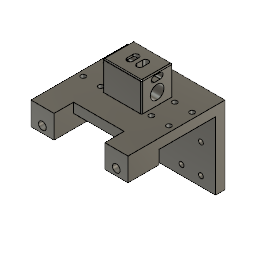
axis_connector (Autodesk Fusion 360 design; units mm, degrees)
Autodesk Fusion 360 part; units mm, degrees
note: some values were not read from the file. Chosen so that the rebuilt part matches the saved one: which bodies a step acts on.
sketch "Sketch1" plane through (0, 0, 0) normal (0, 0, 1) x (1, 0, 0)
  line L0 (0, 0) -> (100, 0)
  line L1 (100, 0) -> (100, 80)
  line L2 (100, 80) -> (0, 80)
  line L3 (0, 80) -> (0, 0)
  dimension "d1" = 80
  dimension "d2" = 100
  constraint horizontal L0
  constraint vertical L1
  constraint horizontal L2
  constraint vertical L3
  constraint coincident L0.start L3.end
  measures "d1" distance of L0.start L2.end
  measures "d2" distance of L0.start L0.end
extrude "Extrude1" add sketch "Sketch1" along normal blind 10 makes body 1
sketch "Sketch2" plane through (0, 0, 10) normal (0, 0, 1) x (-1, 0, 0)
  line L0 (0, -80) -> (0, 0)
  line L1 (0, 0) -> (-100, 0)
  line L2 (-100, 0) -> (-100, -80)
  line L3 (-100, -80) -> (0, -80)
  line L4 (-30, -40) -> (-30, -55.875)
  line L5 (-30, -55.875) -> (0, -55.875)
  line L6 (0, -55.875) -> (0, -40)
  line L7 (-30.0062, -40) -> (-30.0062, -24.125)
  line L8 (-30.0062, -24.125) -> (0, -24.125)
  line L9 (0, -24.125) -> (0, -40)
  line L10 (-70, -40) -> (-70, -55.875)
  line L11 (-70, -55.875) -> (-100, -55.875)
  line L12 (-100, -55.875) -> (-100, -40)
  line L13 (-70, -40) -> (-70, -24.125)
  line L14 (-70, -24.125) -> (-100, -24.125)
  line L15 (-100, -24.125) -> (-100, -40)
  line L16 (0, -40) -> (-30, -40)
  line L17 (-30, -40) -> (-30, -28)
  line L18 (0, -28) -> (0, -40)
  line L19 (0, -40) -> (-30, -40)
  line L20 (-30, -40) -> (-30, -52)
  line L21 (0, -52) -> (0, -40)
  line L22 (-6, -54.5) -> (-6, -55.875)
  line L23 (-24, -54.5) -> (-24, -55.875)
  circle A0 centre (-6, -52) radius 2.5
  circle A1 centre (-24, -52) radius 2.5
  line L24 (-6, -25.5) -> (-6, -24.125)
  line L25 (-24.0062, -25.5) -> (-24.0062, -24.125)
  circle A2 centre (-6, -28) radius 2.5
  circle A3 centre (-24.0062, -28) radius 2.5
  line L26 (-30, -28) -> (-26.5062, -28)
  line L27 (-21.5062, -28) -> (-8.5, -28)
  line L28 (-3.5, -28) -> (0, -28)
  line L29 (-3.5, -52) -> (0, -52)
  line L30 (-30, -52) -> (-26.5, -52)
  line L31 (-21.5, -52) -> (-8.5, -52)
  line L32 (-100, -40) -> (-70, -40)
  line L33 (-70, -40) -> (-70, -52)
  line L34 (-100, -52) -> (-100, -40)
  line L35 (-100, -40) -> (-70, -40)
  line L36 (-70, -40) -> (-70, -28)
  line L37 (-100, -28) -> (-100, -40)
  line L38 (-76, -25.5079) -> (-76, -24.125)
  line L39 (-94, -25.5) -> (-94, -24.125)
  line L40 (-76, -54.5) -> (-76, -55.875)
  line L41 (-94, -54.5) -> (-94, -55.875)
  circle A4 centre (-94, -28) radius 2.5
  circle A5 centre (-76, -52) radius 2.5
  circle A6 centre (-94, -52) radius 2.5
  line L42 (-70, -28) -> (-73.6983, -28)
  line L43 (-78.6983, -28) -> (-91.5, -28)
  line L44 (-96.5, -28) -> (-100, -28)
  line L45 (-70, -52) -> (-73.5, -52)
  line L46 (-78.5, -52) -> (-91.5, -52)
  line L47 (-96.5, -52) -> (-100, -52)
  line L48 (-30, -40) -> (-70, -40)
  line L49 (-78.5, -28) -> (-78.6983, -28)
  circle A7 centre (-76, -28) radius 2.5
  line L50 (-30, -24) -> (-70, -24)
  line L51 (-70, -24) -> (-70, -56)
  line L52 (-70, -56) -> (-30, -56)
  line L53 (-30, -56) -> (-30, -24)
  line L54 (-30, -24) -> (-70, -56) construction
  line L55 (-70, -24) -> (-30, -56) construction
  point P0 (0, -40)
  point P1 (-100, -40)
  point P2 (-50, -40)
  point P3 (-50, -40)
  dimension "d5" = 15.875
  dimension "d6" = 30
  dimension "d7" = 15.875
  dimension "d8" = 30
  dimension "d9" = 15.875
  dimension "d10" = 15.875
  dimension "d11" = 30
  dimension "d12" = 12
  dimension "d13" = 12
  dimension "d15" = 6
  dimension "d16" = 6
  dimension "d17" = 5
  dimension "d18" = 5
  dimension "d19" = 6
  dimension "d20" = 6
  dimension "d21" = 5
  dimension "d22" = 5
  dimension "d24" = 12
  dimension "d25" = 30
  dimension "d26" = 12
  dimension "d27" = 6
  dimension "d28" = 6
  dimension "d29" = 6
  dimension "d30" = 6
  dimension "d32" = 5
  dimension "d33" = 5
  dimension "d34" = 5
  dimension "d35" = 30
  dimension "d36" = 5
  dimension "d37" = 32
  dimension "d38" = 40
  constraint midpoint L0 P0
  constraint midpoint L2 P1
  constraint vertical L4
  constraint horizontal L5
  constraint vertical L6
  constraint coincident P0 L6.end
  constraint vertical L7
  constraint horizontal L8
  constraint vertical L9
  constraint vertical L10
  constraint horizontal L11
  constraint vertical L12
  constraint coincident P1 L12.end
  constraint vertical L13
  constraint horizontal L14
  constraint vertical L15
  constraint horizontal L16
  constraint vertical L17
  constraint horizontal L26
  constraint vertical L18
  constraint horizontal L19
  constraint vertical L20
  constraint horizontal L30
  constraint vertical L21
  constraint coincident L5 L22.end
  constraint perpendicular L5 L22
  constraint coincident L5 L23.end
  constraint perpendicular L5 L23
  constraint coincident L8 L24.end
  constraint perpendicular L8 L24
  constraint coincident L8 L25.end
  constraint perpendicular L8 L25
  constraint coincident A2 L24.start
  constraint coincident A3 L25.start
  constraint coincident A3 L26.end
  constraint coincident A3 L27.start
  constraint collinear L26 L27
  constraint coincident A2 L27.end
  constraint coincident A2 L28.start
  constraint collinear L27 L28
  constraint coincident A0 L29.start
  constraint collinear L29 L30
  constraint coincident A0 L31.end
  constraint coincident A0 L22.start
  constraint coincident A1 L31.start
  constraint collinear L30 L31
  constraint coincident A1 L30.end
  constraint coincident A1 L23.start
  constraint horizontal L32
  constraint vertical L33
  constraint horizontal L45
  constraint vertical L34
  constraint horizontal L35
  constraint vertical L36
  constraint horizontal L42
  constraint vertical L37
  constraint coincident L14 L38.end
  constraint perpendicular L14 L38
  constraint coincident L14 L39.end
  constraint perpendicular L14 L39
  constraint coincident L11 L40.end
  constraint perpendicular L11 L40
  constraint coincident L11 L41.end
  constraint perpendicular L11 L41
  constraint collinear L42 L43
  constraint coincident A4 L43.end
  constraint collinear L43 L44
  constraint coincident A4 L39.start
  constraint coincident A4 L44.start
  constraint coincident A5 L45.end
  constraint collinear L45 L46
  constraint coincident A5 L40.start
  constraint coincident A5 L46.start
  constraint coincident A6 L46.end
  constraint collinear L46 L47
  constraint coincident A6 L41.start
  constraint coincident A6 L47.start
  constraint perpendicular L36 L48
  constraint parallel L43 L49
  constraint coincident A7 L49.start
  constraint midpoint L48 P3
  constraint perpendicular L50 L51
  constraint parallel L50 L52
  constraint parallel L51 L53
  constraint horizontal L50
  constraint coincident L54 P3
  constraint coincident L55 P3
  constraint coincident P3 P2
  measures "d5" distance of P0 L5.end
  measures "d6" distance of P0 L4.start
  measures "d7" distance of P0 L8.end
  measures "d8" distance of P1 L10.start
  measures "d9" distance of P1 L11.end
  measures "d10" distance of P1 L14.end
  measures "d11" distance of P0 L4.start
  measures "d12" distance of P0 L18.start
  measures "d13" distance of P0 L21.start
  measures "d15" distance of L6 L22
  measures "d16" distance of L4 L23
  measures "d17" diameter of A0
  measures "d18" diameter of A1
  measures "d19" distance of L9 L24
  measures "d20" distance of L7 L25
  measures "d21" diameter of A2
  measures "d22" diameter of A3
  measures "d24" distance of P1 L34.start
  measures "d25" distance of P1 L10.start
  measures "d26" distance of P1 L37.start
  measures "d27" distance of L10 L40
  measures "d28" distance of L12 L41
  measures "d29" distance of L13 L38
  measures "d30" distance of L15 L39
  measures "d32" diameter of A4
  measures "d33" diameter of A5
  measures "d34" diameter of A6
  measures "d35" distance of L13 L37
  measures "d36" diameter of A7
  measures "d37" distance of L50.end L51.end
  measures "d38" distance of L51.end L52.end
extrude "Extrude2" cut sketch "Sketch2" against normal blind 10 contours A0 | A1 | A6 | A2 | A5 | A3 | A4 | A7 bodies 1
sketch "Sketch3" plane through (0, 0, 10) normal (0, 0, 1) x (-1, 0, 0)
  circle A0 centre (-94, -52) radius 2.5
  circle A1 centre (-24.0062, -28) radius 2.5
  circle A2 centre (-6, -28) radius 2.5
  circle A3 centre (-76, -28) radius 2.5
  circle A4 centre (-76, -52) radius 2.5
  circle A5 centre (-24, -52) radius 2.5
  circle A6 centre (-6, -52) radius 2.5
  circle A7 centre (-94, -28) radius 2.5
  line L0 (0, -80) -> (0, 0)
  line L1 (0, 0) -> (-100, 0)
  line L2 (-100, 0) -> (-100, -80)
  line L3 (-100, -80) -> (0, -80)
  line L4 (-70, -56) -> (-30, -56)
  line L5 (-30, -56) -> (-30, -24)
  line L6 (-30, -24) -> (-70, -24)
  line L7 (-70, -24) -> (-70, -56)
  line L8 (-70, -56) -> (-30, -24) construction
  line L9 (-30, -56) -> (-70, -24) construction
  line L10 (0, -40) -> (-30, -40)
  line L11 (-70, -40) -> (-100, -40)
  dimension "d41" = 32
  dimension "d42" = 40
  constraint midpoint L0 L10.start
  constraint midpoint L2 L11.end
  constraint perpendicular L4 L5
  constraint parallel L4 L6
  constraint parallel L5 L7
  constraint horizontal L4
  constraint coincident L5 L10.end
  constraint collinear L10 L11
  constraint coincident L7 L11.start
  measures "d41" distance of L4.end L5.end
  measures "d42" distance of L5.end L6.end
extrude "Extrude3" add sketch "Sketch3" along normal blind 30 contours L4 L5 L6 L7 bodies 1
sketch "Sketch4" plane through (70, 0, 0) normal (1, 0, 0) x (0, 1, 0)
  line L0 (24, 10) -> (56, 10)
  line L1 (56, 10) -> (56, 40)
  line L2 (56, 40) -> (24, 40)
  line L3 (24, 40) -> (24, 10)
  line L4 (24, 10) -> (40, 10)
  line L5 (40, 10) -> (40, 15)
  line L6 (33, 22) -> (24, 22)
  line L7 (24, 22) -> (24, 10)
  circle A0 centre (40, 22) radius 7
  dimension "d45" = 12
  dimension "d46" = 14
  constraint horizontal L4
  constraint vertical L5
  constraint horizontal L6
  constraint vertical L7
  constraint coincident L0.start L3.end
  constraint coincident A0 L5.end
  constraint coincident A0 L6.start
  measures "d45" distance of L0.start L6.end
  measures "d46" diameter of A0
extrude "Extrude4" cut sketch "Sketch4" against normal blind 40 contours A0 bodies 1
sketch "Sketch5" plane through (0, 0, 0) normal (0, 0, -1) x (1, 0, 0)
  circle A0 centre (94, -52) radius 2.5
  circle A1 centre (24.0062, -28) radius 2.5
  circle A2 centre (6, -28) radius 2.5
  circle A3 centre (76, -28) radius 2.5
  circle A4 centre (76, -52) radius 2.5
  circle A5 centre (24, -52) radius 2.5
  circle A6 centre (6, -52) radius 2.5
  circle A7 centre (94, -28) radius 2.5
  line L0 (0, 0) -> (0, -80)
  line L1 (0, -80) -> (100, -80)
  line L2 (100, -80) -> (100, 0)
  line L3 (100, 0) -> (0, 0)
  line L4 (0, 0) -> (24, 0)
  line L5 (24, 0) -> (24, -20)
  line L6 (24, -20) -> (0, -20)
  line L7 (0, -20) -> (0, 0)
  line L8 (100, 0) -> (76, 0)
  line L9 (76, 0) -> (76, -20)
  line L10 (76, -20) -> (100, -20)
  line L11 (100, -20) -> (100, 0)
  point P0 (50, -80)
  point P1 (50, -70)
  dimension "d49" = 24
  dimension "d50" = 20
  constraint midpoint L1 P0
  constraint horizontal L4
  constraint vertical L5
  constraint horizontal L6
  constraint vertical L7
  constraint coincident L0.start L3.end
  constraint horizontal L8
  constraint vertical L9
  constraint horizontal L10
  constraint vertical L11
  constraint coincident L2.end L3.start
  measures "d49" distance of L2.end L8.end
  measures "d50" distance of L2.end L10.end
sketch "Sketch6" plane through (0, 0, 0) normal (0, -1, 0) x (1, 0, 0)
  line L0 (0, 0) -> (100, 0)
  line L1 (100, 0) -> (100, 10)
  line L2 (100, 10) -> (0, 10)
  line L3 (0, 10) -> (0, 0)
  line L4 (0, 10) -> (24, 10)
  line L5 (24, 10) -> (24, 0)
  line L6 (24, 0) -> (0, 0)
  line L7 (0, 0) -> (0, 10)
  line L8 (100, 10) -> (76, 10)
  line L9 (76, 10) -> (76, 0)
  line L10 (76, 0) -> (100, 0)
  line L11 (100, 0) -> (100, 10)
  point P0 (24, 0)
  dimension "d51" = 24
  constraint horizontal L4
  constraint vertical L5
  constraint horizontal L6
  constraint vertical L7
  constraint coincident P0 L5.end
  constraint coincident L2.end L3.start
  constraint horizontal L8
  constraint vertical L9
  constraint horizontal L10
  constraint vertical L11
  constraint coincident L1.end L2.start
  measures "d51" distance of L1.end L8.end
extrude "Extrude5" add sketch "Sketch6" along normal blind 20 contours L0 L2 L3 L4 L5 L6 L7 | L0 L1 L2 L8 L9 L10 L11 bodies 1
sketch "Sketch7" plane through (0, 0, 0) normal (0, 0, -1) x (1, 0, 0)
  line L0 (0, 20) -> (24, 20)
  line L1 (24, 20) -> (24, 0)
  line L2 (24, 0) -> (0, 0)
  line L3 (0, 0) -> (0, 20)
  line L4 (100, 0) -> (76, 0)
  line L5 (76, 0) -> (76, 20)
  line L6 (76, 20) -> (100, 20)
  line L7 (100, 20) -> (100, 0)
  point P0 (0, 20)
  point P1 (24, 0)
  point P2 (100, 0)
  point P3 (76, 20)
  constraint horizontal L0
  constraint vertical L1
  constraint horizontal L2
  constraint vertical L3
  constraint coincident P1 L1.end
  constraint coincident P0 L0.start
  constraint horizontal L4
  constraint vertical L5
  constraint horizontal L6
  constraint vertical L7
  constraint coincident P3 L5.end
  constraint coincident P2 L4.start
extrude "Extrude6" add sketch "Sketch7" sketch "Sketch5" along normal blind 14 of sketch 2 contours L0 L3 L4 L5 L6 L7 | L2 L3 L8 L9 L10 L11 bodies 1
sketch "Sketch8" plane through (0, 0, 0) normal (0, 0, -1) x (1, 0, 0)
  line L0 (76, -20) -> (76, 0)
  line L1 (76, 0) -> (24, 0)
  line L2 (24, 0) -> (24, -20)
  line L3 (24, -20) -> (0, -20)
  line L4 (0, -20) -> (0, -80)
  line L5 (0, -80) -> (100, -80)
  line L6 (100, -80) -> (100, -20)
  line L7 (100, -20) -> (76, -20)
  circle A0 centre (94, -28) radius 2.5
  circle A1 centre (6, -52) radius 2.5
  circle A2 centre (24, -52) radius 2.5
  circle A3 centre (76, -52) radius 2.5
  circle A4 centre (76, -28) radius 2.5
  circle A5 centre (6, -28) radius 2.5
  circle A6 centre (24.0062, -28) radius 2.5
  circle A7 centre (94, -52) radius 2.5
  line L8 (0, -80) -> (100, -80)
  line L9 (100, -80) -> (100, -70)
  line L10 (100, -70) -> (0, -70)
  line L11 (0, -70) -> (0, -80)
  constraint horizontal L8
  constraint vertical L9
  constraint horizontal L10
  constraint vertical L11
  constraint coincident L6 L9.end
  constraint coincident L4.end L5.start
extrude "Extrude7" add sketch "Sketch8" along normal blind 50 separate body contours L4 L5 L6 L8 L9 L10 L11 makes body 2
sketch "Sketch9" plane through (0, -20, 0) normal (0, -1, 0) x (1, 0, 0)
  line L0 (24, -14) -> (24, 10)
  line L1 (24, 10) -> (0, 10)
  line L2 (0, 10) -> (0, -14)
  line L3 (0, -14) -> (24, -14)
  line L4 (0, 0) -> (0, -14)
  circle A0 centre (12, -7) radius 4
  line L5 (12, 10) -> (12, -3)
  line L6 (12, -11) -> (12, -14)
  line L7 (0, -7) -> (8, -7)
  line L8 (16, -7) -> (24, -7)
  dimension "d58" = 8
  constraint midpoint L1 L5.start
  constraint midpoint L3 L6.end
  constraint midpoint L4 L7.start
  constraint coincident L0 L8.end
  constraint coincident A0 L6.start
  constraint collinear L5 L6
  constraint coincident A0 L8.start
  constraint collinear L7 L8
  constraint coincident A0 L5.end
  constraint coincident A0 L7.end
  measures "d58" diameter of A0
extrude "Extrude8" cut sketch "Sketch9" against normal blind 40 contours A0 bodies 1
sketch "Sketch10" plane through (0, -20, 0) normal (0, -1, 0) x (1, 0, 0)
  line L0 (100, -14) -> (100, 10)
  line L1 (100, 10) -> (76, 10)
  line L2 (76, 10) -> (76, -14)
  line L3 (76, -14) -> (100, -14)
  line L4 (100, 0) -> (100, -14)
  line L5 (76, 0) -> (76, -14)
  circle A0 centre (88, -7) radius 4
  line L6 (100, -7) -> (92, -7)
  line L7 (84, -7) -> (76, -7)
  line L8 (88, 10) -> (88, -3)
  line L9 (88, -11) -> (88, -14)
  dimension "d61" = 8
  constraint midpoint L1 L8.start
  constraint midpoint L3 L9.end
  constraint midpoint L4 L6.start
  constraint midpoint L5 L7.end
  constraint coincident A0 L7.start
  constraint collinear L6 L7
  constraint coincident A0 L8.end
  constraint collinear L8 L9
  constraint coincident A0 L6.end
  constraint coincident A0 L9.start
  measures "d61" diameter of A0
extrude "Extrude9" cut sketch "Sketch10" against normal blind 40 contours A0 bodies 1
sketch "Sketch11" plane through (70, 0, 0) normal (1, 0, 0) x (0, 1, 0)
  circle A0 centre (40, 22) radius 7
  line L0 (24, 10) -> (56, 10)
  line L1 (56, 10) -> (56, 40)
  line L2 (56, 40) -> (24, 40)
  line L3 (24, 40) -> (24, 10)
  line L4 (24, 40) -> (56, 40)
  line L5 (56, 40) -> (56, 30)
  line L6 (56, 30) -> (24, 30)
  line L7 (24, 30) -> (24, 40)
  line L8 (37, 32) -> (43, 32)
  arc A1 (43, 32) -> (43, 38) centre (43, 35) ccw
  line L9 (43, 38) -> (37, 38)
  arc A2 (37, 38) -> (37, 32) centre (37, 35) ccw
  line L10 (37, 35) -> (43, 35) construction
  line L11 (40, 40) -> (40, 38)
  line L12 (40, 32) -> (40, 30)
  point P0 (40, 40)
  dimension "d64" = 32
  dimension "d65" = 6
  constraint midpoint L2 P0
  constraint horizontal L4
  constraint vertical L5
  constraint horizontal L6
  constraint vertical L7
  constraint coincident L2.end L3.start
  constraint coincident P0 L11.start
  constraint midpoint L6 L12.end
  constraint tangent L8 A1
  constraint tangent A1 L9
  constraint parallel L8 L9
  constraint tangent L9 A2
  constraint tangent L8 A2
  constraint perpendicular L10 L11
  constraint coincident L8 L12.start
  constraint collinear L11 L12
  constraint coincident L9 L11.end
  measures "d64" distance of L2.end L1.end
  measures "d65" diameter of A1
extrude "Extrude10" cut sketch "Sketch11" against normal blind 15 contours L8 A1 L9 A2 bodies 1
sketch "Sketch12" plane through (0, 0, 40) normal (0, 0, 1) x (-1, 0, 0)
  line L0 (-70, -24) -> (-70, -56)
  line L1 (-70, -56) -> (-30, -56)
  line L2 (-30, -56) -> (-30, -24)
  line L3 (-30, -24) -> (-70, -24)
  line L4 (-70, -56) -> (-55, -56)
  line L5 (-55, -24) -> (-70, -24)
  line L6 (-70, -24) -> (-70, -56)
  line L7 (-30, -56) -> (-45, -56)
  line L8 (-45, -24) -> (-30, -24)
  line L9 (-30, -24) -> (-30, -56)
  line L10 (-58, -37) -> (-58, -43)
  arc A0 (-58, -43) -> (-52, -43) centre (-55, -43) ccw
  line L11 (-52, -43) -> (-52, -37)
  arc A1 (-52, -37) -> (-58, -37) centre (-55, -37) ccw
  line L12 (-48, -37) -> (-48, -43)
  arc A2 (-48, -43) -> (-42, -43) centre (-45, -43) ccw
  line L13 (-42, -43) -> (-42, -37)
  arc A3 (-42, -37) -> (-48, -37) centre (-45, -37) ccw
  line L14 (-55, -56) -> (-55, -46)
  line L15 (-55, -34) -> (-55, -24)
  line L16 (-45, -56) -> (-45, -46)
  line L17 (-45, -34) -> (-45, -24)
  point P0 (-55, -43)
  point P1 (-45, -40)
  dimension "d68" = 6
  constraint horizontal L4
  constraint vertical L14
  constraint horizontal L5
  constraint vertical L6
  constraint coincident L3 L5.start
  constraint coincident L0.end L1.start
  constraint horizontal L7
  constraint vertical L16
  constraint horizontal L8
  constraint vertical L9
  constraint coincident L3 L8.start
  constraint coincident L1.end L2.start
  constraint tangent L10 A0
  constraint tangent A0 L11
  constraint parallel L10 L11
  constraint tangent L11 A1
  constraint tangent L10 A1
  constraint coincident P0 A0.centre
  constraint tangent L12 A2
  constraint tangent A2 L13
  constraint parallel L12 L13
  constraint tangent L13 A3
  constraint tangent L12 A3
  constraint coincident A2.centre L16
  constraint coincident A1 L15.start
  constraint collinear L14 L15
  constraint coincident A0 L14.end
  constraint coincident A2 L16.end
  constraint coincident A3 L17.start
  constraint collinear L16 L17
  constraint coincident P1 L16
  measures "d68" diameter of A2
extrude "Extrude11" cut sketch "Sketch12" against normal blind 8 contours L10 A0 L11 A1 | L12 A2 L13 A3 bodies 1
sketch "Sketch13" plane through (30, 0, 0) normal (-1, 0, 0) x (0, -1, 0)
  circle A0 centre (-40, 22) radius 7
  line L0 (-56, 10) -> (-24, 10)
  line L1 (-24, 10) -> (-24, 40)
  line L2 (-24, 40) -> (-56, 40)
  line L3 (-56, 40) -> (-56, 10)
  line L4 (-56, 40) -> (-24, 40)
  line L5 (-24, 40) -> (-24, 35)
  line L6 (-56, 35) -> (-56, 40)
  line L7 (-43, 32) -> (-37, 32)
  arc A1 (-37, 32) -> (-37, 38) centre (-37, 35) ccw
  line L8 (-37, 38) -> (-43, 38)
  arc A2 (-43, 38) -> (-43, 32) centre (-43, 35) ccw
  line L9 (-24, 35) -> (-34, 35)
  line L10 (-46, 35) -> (-56, 35)
  point P0 (-40, 35)
  dimension "d71" = 32
  dimension "d72" = 5
  dimension "d73" = 6
  constraint horizontal L4
  constraint vertical L5
  constraint horizontal L9
  constraint vertical L6
  constraint coincident L2.end L3.start
  constraint tangent L7 A1
  constraint tangent A1 L8
  constraint parallel L7 L8
  constraint tangent L8 A2
  constraint tangent L7 A2
  constraint coincident A1.centre L9
  constraint coincident A1 L9.end
  constraint coincident A2 L10.start
  constraint collinear L9 L10
  constraint coincident P0 L9
  measures "d71" distance of L2.end L1.end
  measures "d72" distance of L2.end L6.start
  measures "d73" diameter of A1
extrude "Extrude12" cut sketch "Sketch13" against normal blind 15 contours L7 A1 L8 A2 bodies 1
sketch "Sketch14" plane through (0, 80, 0) normal (0, 1, 0) x (-1, 0, 0)
  line L0 (0, 0) -> (-100, 0)
  line L1 (-100, 0) -> (-100, -50)
  line L2 (-100, -50) -> (0, -50)
  line L3 (0, -50) -> (0, 0)
  line L4 (-100, -25) -> (-50, -25)
  line L5 (-50, -25) -> (-50, 0)
  line L6 (-50, 0) -> (-100, 0)
  line L7 (-100, 0) -> (-100, -25)
  line L8 (-100, -25) -> (-50, -25)
  line L9 (-50, -25) -> (-50, -50)
  line L10 (-50, -50) -> (-100, -50)
  line L11 (-100, -50) -> (-100, -25)
  circle A0 centre (-85, -40) radius 2.5
  circle A1 centre (-85, -10) radius 2.5
  circle A2 centre (-65, -10) radius 2.5
  circle A3 centre (-65, -40) radius 2.5
  line L12 (-100, -40) -> (-87.5, -40)
  line L13 (-82.5, -40) -> (-67.5, -40)
  line L14 (-62.5, -40) -> (-50, -40)
  line L15 (-100, -10) -> (-87.5, -10)
  line L16 (-82.5, -10) -> (-67.5, -10)
  line L17 (-62.5, -10) -> (-50, -10)
  dimension "d76" = 25
  dimension "d78" = 25
  dimension "d79" = 10
  dimension "d80" = 10
  dimension "d81" = 5
  dimension "d82" = 5
  dimension "d83" = 5
  dimension "d84" = 5
  constraint horizontal L4
  constraint vertical L5
  constraint horizontal L6
  constraint vertical L7
  constraint midpoint L1 L4.start
  constraint horizontal L8
  constraint vertical L9
  constraint horizontal L10
  constraint vertical L11
  constraint coincident L1 L15.start
  constraint coincident L5 L17.end
  constraint perpendicular L5 L15
  constraint coincident L11 L12.start
  constraint coincident L9 L14.end
  constraint perpendicular L9 L12
  constraint coincident A0.centre L12
  constraint coincident A1.centre L15
  constraint coincident A2.centre L15
  constraint coincident A3.centre L12
  constraint coincident A0 L12.end
  constraint coincident A0 L13.start
  constraint collinear L12 L13
  constraint coincident A3 L13.end
  constraint coincident A3 L14.start
  constraint collinear L13 L14
  constraint coincident A1 L15.end
  constraint coincident A1 L16.start
  constraint collinear L15 L16
  constraint coincident A2 L16.end
  constraint coincident A2 L17.start
  constraint collinear L16 L17
  measures "d76" distance of L4.start L0.end
  measures "d78" distance of L4.start L1.end
  measures "d79" distance of L6 L15
  measures "d80" distance of L10 L12
  measures "d81" diameter of A0
  measures "d82" diameter of A1
  measures "d83" diameter of A2
  measures "d84" diameter of A3
extrude "Extrude13" cut sketch "Sketch14" against normal blind 40 contours A2 | A1 | A3 | A0 bodies 2
combine "Combine1" operation add target body 2 tool bodies 1
fillet "Fillet1" radius 1 8 edges at (70, 40, 40) (70, 24, 25) (70, 56, 25) (50, 24, 40) (50, 56, 40) (30, 24, 25) (30, 40, 40) (30, 56, 25) on bodies 2
sketch "Sketch15" plane through (0, 0, 10) normal (0, 0, 1) x (-1, 0, 0)
  line L0 (-69, -24) -> (-31, -24)
  arc A0 (-30, -25) -> (-31, -24) centre (-31, -25) ccw
  line L1 (-30, -25) -> (-30, -55)
  arc A1 (-31, -56) -> (-30, -55) centre (-31, -55) ccw
  line L2 (-31, -56) -> (-69, -56)
  arc A2 (-70, -55) -> (-69, -56) centre (-69, -55) ccw
  line L3 (-70, -55) -> (-70, -25)
  arc A3 (-69, -24) -> (-70, -25) centre (-69, -25) ccw
  circle A4 centre (-94, -52) radius 2.5
  circle A5 centre (-24.0062, -28) radius 2.5
  circle A6 centre (-6, -28) radius 2.5
  circle A7 centre (-76, -28) radius 2.5
  circle A8 centre (-76, -52) radius 2.5
  circle A9 centre (-24, -52) radius 2.5
  circle A10 centre (-6, -52) radius 2.5
  circle A11 centre (-94, -28) radius 2.5
  line L4 (0, -80) -> (0, 20)
  line L5 (0, 20) -> (-24, 20)
  line L6 (-76, 0) -> (-76, 20)
  line L7 (-76, 20) -> (-100, 20)
  line L8 (-100, 20) -> (-100, -80)
  line L9 (-100, -80) -> (0, -80)
sketch "Sketch16" plane through (0, -20, 0) normal (0, -1, 0) x (1, 0, 0)
  circle A0 centre (12, -7) radius 4
  line L0 (24, -14) -> (24, 10)
  line L1 (24, 10) -> (0, 10)
  line L2 (0, 10) -> (0, -14)
  line L3 (0, -14) -> (24, -14)
sketch "Sketch17" plane through (0, -20, 0) normal (0, -1, 0) x (1, 0, 0)
sketch "Sketch18" plane through (0, 0, -14) normal (0, 0, -1) x (1, 0, 0)
  line L0 (100, 20) -> (76, 20)
  line L1 (76, 20) -> (76, -20)
  line L2 (76, -20) -> (100, -20)
  line L3 (100, -20) -> (100, 20)
  line L4 (76, -20) -> (100, -20)
  line L5 (100, -20) -> (100, -12)
  line L6 (100, -12) -> (76, -12)
  line L7 (76, -12) -> (76, -20)
  dimension "d88" = 8
  constraint horizontal L4
  constraint vertical L5
  constraint horizontal L6
  constraint vertical L7
  constraint coincident L1.end L2.start
  measures "d88" distance of L1.end L6.end
extrude "Extrude14" cut sketch "Sketch18" against normal blind 14 contours L1 L2 L3 L4 L5 L6 L7 bodies 2
sketch "Sketch19" plane through (0, -20, 0) normal (0, -1, 0) x (1, 0, 0)
  line L0 (100, -14) -> (100, 10)
  line L1 (100, 10) -> (76, 10)
  line L2 (76, 10) -> (76, -14)
  line L3 (76, -14) -> (100, -14)
split "Split1" by plane through (0, 0, 0) normal (0, 0, -1) bodies 2 makes body 3 at (20.9159, 80, -20.3616) makes body 4 at (88.4974, -9.3333, -10.969) makes body 5 at (15.9801, -6.6667, -6.6017)
move_body "Move1" bodies 3 to x (1, 0, 0) y (0, 1, 0) z (0, 0, 1) at (-0.097, 0.1553, -18.1207)
move_body "Move2" bodies 3 to x (1, 0, 0) y (0, 1, 0) z (0, 0, 1) at (-0.5514, 70.88, 15.1553)
sketch "Sketch20" plane through (0, 0, 0) normal (0, 0, -1) x (1, 0, 0)
  circle A0 centre (94, -52) radius 2.5
  circle A1 centre (24.0062, -28) radius 2.5
  circle A2 centre (6, -28) radius 2.5
  circle A3 centre (76, -28) radius 2.5
  circle A4 centre (76, -52) radius 2.5
  circle A5 centre (24, -52) radius 2.5
  circle A6 centre (6, -52) radius 2.5
  circle A7 centre (94, -28) radius 2.5
  line L0 (100, -80) -> (100, 20)
  line L1 (100, 20) -> (76, 20)
  line L2 (76, 20) -> (76, 0)
  line L3 (76, 0) -> (24, 0)
  line L4 (24, 0) -> (24, 20)
  line L5 (24, 20) -> (0, 20)
  line L6 (0, 20) -> (0, -80)
  line L7 (0, -80) -> (100, -80)
  line L8 (0, -80) -> (100, -80)
  line L9 (100, -80) -> (100, -70)
  line L10 (100, -70) -> (0, -70)
  line L11 (0, -70) -> (0, -80)
  dimension "d91" = 100
  dimension "d92" = 10
  constraint horizontal L8
  constraint vertical L9
  constraint horizontal L10
  constraint vertical L11
  constraint coincident L6.end L7.start
  measures "d91" distance of L6.end L0.start
  measures "d92" distance of L6.end L10.end
extrude "Extrude15" add sketch "Sketch20" along normal blind 20 contours L0 L6 L7 L8 L9 L10 L11 bodies 2
move_body "Align1" bodies 3 to x (1, 0, 0) y (0, 1, 0) z (0, 0, 1) at (0, 0, -17.0346)
move_face "MoveFace1" by (0, -10, 0) 1 faces at (-0.6484, 144.3686, -36.6667) on bodies 3
combine "Combine2" operation add target body 4 tool bodies 5 2
move_body "Align2" bodies 4 to x (1, 0, 0) y (0, 1, 0) z (0, 0, 1) at (-0.6484, 71.0353, 0)
combine "Combine3" operation add target body 4 tool bodies 3
sketch "Sketch21" plane through (0, 141.0353, 0) normal (0, -1, 0) x (1, 0, 0)
  circle A0 centre (64.3516, -60) radius 2.5
  circle A1 centre (84.3516, -30) radius 2.5
  circle A2 centre (84.3516, -60) radius 2.5
  circle A3 centre (64.3516, -30) radius 2.5
  line L0 (99.3516, 0) -> (-0.6484, 0)
  line L1 (-0.6484, 0) -> (-0.6484, -70)
  line L2 (-0.6484, -70) -> (99.3516, -70)
  line L3 (99.3516, -70) -> (99.3516, 0)
  line L4 (64.3516, -30) -> (64.3516, -60)
  line L5 (64.3516, -60) -> (84.3516, -60)
  line L6 (84.3516, -60) -> (84.3516, -30)
  line L7 (84.3516, -30) -> (64.3516, -30)
  line L8 (84.3516, -45) -> (-0.7565, -45)
  line L9 (100, 0) -> (0, 0)
  dimension "d95" = 45
  constraint coincident A3.centre L4.start
  constraint coincident A0.centre L4.end
  constraint coincident A2.centre L5.end
  constraint coincident A1.centre L6.end
  constraint midpoint L6 L8.start
  constraint perpendicular L1 L8
  measures "d95" distance of L8 L9
sketch "Sketch22" plane through (0, 51.0353, 0) normal (0, -1, 0) x (1, 0, 0)
  line L0 (-0.6484, 10) -> (-0.6484, -14)
  line L1 (-0.6484, -14) -> (23.3516, -14)
  line L2 (23.3516, -14) -> (23.3516, 10)
  line L3 (23.3516, 10) -> (-0.6484, 10)
  circle A0 centre (11.3516, -7) radius 4
  line L4 (0, 10) -> (24, 10)
  line L5 (100, 0) -> (0, 0)
  dimension "d96" = 17
  dimension "d97" = 7
  measures "d96" distance of A0.centre L4
  measures "d97" distance of A0.centre L5
